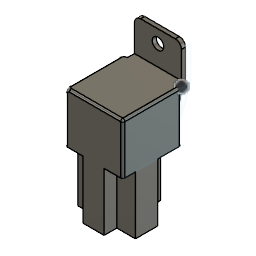
relay_jd2912_v0_1 (Autodesk Fusion 360 design; units mm, degrees)
part number: 2026-05-28-16-02-39-412
Autodesk Fusion 360 part; units mm, degrees
box "长方体基本要素1" add length 28.3 width 27.7 height 24.5 placed x (0, 0, 1) y (1, 0, 0) z (0, 1, 0) at (0, 0, 0)
sketch "草图2" plane through (27.7, 0, 0) normal (1, 0, 0) x (0, 0, -1)
  line L0 (-28.3, 24.5) -> (-28.3, 0)
  line L1 (-28.3, 0) -> (0, 0)
  line L2 (0, 0) -> (0, 24.5)
  line L3 (0, 24.5) -> (-28.3, 24.5)
  line L4 (0, 24.5) -> (4.5, 24.5)
  line L5 (0, 24.5) -> (0, 11.5)
  line L6 (4.5, 24.5) -> (0, 11.5)
  line L7 (4.5, 24.5) -> (2.5, 24.5)
  line L8 (2.5, 24.5) -> (2.5, 40.5)
  line L9 (4.5, 24.5) -> (4.5, 40.5)
  line L10 (2.5, 40.5) -> (4.5, 40.5)
  dimension "d8" = 4.5
  dimension "d9" = 13
  dimension "d10" = 2
  dimension "d11" = 16
  constraint coincident L2.end L3.start
  constraint perpendicular L2 L4
  constraint perpendicular L4 L5
  constraint parallel L4 L7
  constraint perpendicular L4 L8
  constraint perpendicular L4 L9
  constraint equal L8 L9
  measures "d8" distance of L2.end L4.end
  measures "d9" distance of L2.end L5.end
  measures "d10" distance of L4.end L7.end
  measures "d11" distance of L7.end L8.end
extrude "拉伸3" add sketch "草图2" against normal blind 25.2 contours L2 L4 L5 L6 L7 | L4 L7 L8 L9 L10
extrude "拉伸4" cut sketch "草图2" against normal blind 2.5 contours L2 L4 L5 L6 L7 | L4 L7 L8 L9 L10
fillet "圆角4" radius 1 6 edges at (26.45, 24.5, 0) (13.85, 24.5, 28.3) (0, 12.25, 28.3) (0, 24.5, 14.15) (0, 12.25, 0) (1.25, 24.5, 0)
fillet "圆角5" radius 1 5 edges at (27.7, 11.75, 28.3) (27.7, 24.2071, 28.0071) (27.7, 24.5, 14.15) (27.7, 24.2071, 0.2929) (27.7, 11.75, 0)
fillet "圆角6" radius 3 2 edges at (25.2, 40.5, -3.5) (2.5, 40.5, -3.5)
fillet "圆角7" radius 2 1 edges at (13.85, 24.5, -4.5)
sketch "草图3" plane through (0, 0, -2.5) normal (0, 0, 1) x (1, 0, 0)
  arc A0 (5.5, 40.5) -> (2.5, 37.5) centre (5.5, 37.5) ccw
  line L0 (2.5, 37.5) -> (2.5, 24.5)
  line L1 (2.5, 24.5) -> (25.2, 24.5)
  line L2 (25.2, 24.5) -> (25.2, 37.5)
  arc A1 (25.2, 37.5) -> (22.2, 40.5) centre (22.2, 37.5) ccw
  line L3 (22.2, 40.5) -> (5.5, 40.5)
  line L4 (13.85, 40.5) -> (13.85, 37) construction
  line L5 (13.85, 37) -> (13.85, 34.25) construction
  circle A2 centre (13.85, 34.25) radius 2.75
  point P0 (13.85, 40.5)
  dimension "d34" = 3.5
  dimension "d35" = 2.75
  dimension "d36" = 5.5
  constraint midpoint L3 P0
  constraint coincident P0 L4.start
  constraint perpendicular L3 L4
  constraint parallel L4 L5
  constraint coincident L5.end A2.centre
  measures "d34" distance of P0 L4.end
  measures "d35" distance of L4.end L5.end
  measures "d36" diameter of A2
extrude "拉伸5" cut sketch "草图3" against normal blind 10 contours A2
sketch "草图4" plane through (0, 0, 0) normal (0, -1, 0) x (1, 0, 0)
  arc A0 (27.7, 27.3) -> (26.7, 28.3) centre (26.7, 27.3) ccw
  line L0 (26.7, 28.3) -> (1, 28.3)
  arc A1 (1, 28.3) -> (0, 27.3) centre (1, 27.3) ccw
  line L1 (0, 27.3) -> (0, 1)
  arc A2 (0, 1) -> (1, 0) centre (1, 1) ccw
  line L2 (1, 0) -> (26.7, 0)
  arc A3 (26.7, 0) -> (27.7, 1) centre (26.7, 1) ccw
  line L3 (27.7, 1) -> (27.7, 27.3)
  line L4 (27.7, 28.3) -> (27.7, 0)
  line L5 (8.5, 28.3) -> (8.5, 22.3)
  line L6 (18.7, 28.3) -> (18.7, 22.2)
  line L7 (27.7, 22.2) -> (18.7, 22.2)
  line L8 (0, 11) -> (9.8, 11)
  line L9 (27.7, 11.4) -> (17.7, 11.4)
  line L10 (17.7, 0) -> (17.7, 11.4)
  line L11 (9.8, 0) -> (9.8, 11)
  line L12 (9.8, 22.2) -> (9.8, 22.3)
  line L13 (0, 22.3) -> (8.5, 22.3)
  point P0 (8.5, 28.3)
  point P1 (18.7, 28.3)
  point P2 (0, 22.3)
  point P3 (0, 11)
  point P4 (9.8, 0)
  point P5 (17.7, 0)
  point P6 (27.7, 11.4)
  point P7 (27.7, 22.2)
  dimension "d39" = 8.5
  dimension "d40" = 9
  dimension "d41" = 6
  dimension "d42" = 11
  dimension "d43" = 9.8
  dimension "d44" = 10
  dimension "d45" = 11.4
  dimension "d46" = 6.1
  constraint coincident L0 P0
  constraint coincident L0 P1
  constraint coincident L1 P2
  constraint coincident L1 P3
  constraint coincident L2 P4
  constraint coincident L2 P5
  constraint coincident L4 P6
  constraint coincident L4 P7
  constraint coincident P2 L13.start
  constraint perpendicular L1 L13
  constraint coincident P0 L5.start
  constraint perpendicular L5 L13
  constraint coincident P1 L6.start
  constraint perpendicular L0 L6
  constraint coincident P7 L7.start
  constraint perpendicular L6 L7
  constraint coincident P3 L8.start
  constraint perpendicular L1 L8
  constraint coincident P6 L9.start
  constraint perpendicular L4 L9
  constraint coincident P5 L10.start
  constraint perpendicular L2 L10
  constraint coincident P4 L11.start
  constraint perpendicular L8 L11
  constraint collinear L11 L12
  measures "d39" distance of L1 P0
  measures "d40" distance of P1 L4
  measures "d41" distance of L0 P2
  measures "d42" distance of L2 P3
  measures "d43" distance of L1 P4
  measures "d44" distance of L3 P5
  measures "d45" distance of L2 P6
  measures "d46" distance of L0 P7
extrude "拉伸6" add sketch "草图4" along normal blind 28 contours L0 L1 L2 L3 L4 L5 L6 L7 L8 L9 L10 L11 L13
extrude "拉伸1" [suppressed]
fillet "圆角1" [suppressed]
fillet "圆角2" [suppressed]
fillet "圆角3" [suppressed]
extrude "拉伸2" [suppressed]
